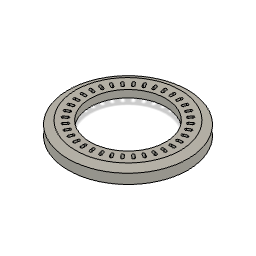
ROTORB (Autodesk Fusion 360 design; units mm, degrees)
Autodesk Fusion 360 part; units mm, degrees
sketch "Sketch1" plane through (0, 0, 0) normal (0, 1, 0) x (1, 0, 0)
  circle A0 centre (0, 0) radius 49.1
  dimension "d1" = 98.2
  constraint coincident A0.centre origin
  measures "d1" diameter of A0
ref_plane "WorkPlane1" through (0, 3, 0) normal (0, 1, 0) x (0, 0, 1)
sketch "Sketch2" plane through (0, 3, 0) normal (0, 1, 0) x (1, 0, 0)
  circle A0 centre (0, 0) radius 43
  dimension "d3" = 86
  constraint coincident A0.centre origin
  measures "d3" diameter of A0
loft "Loft1" add profiles "Sketch1", "Sketch2" section 1 section 2
sketch "Sketch3" plane through (0, 3, 0) normal (0, 1, 0) x (-1, 0, 0)
  circle A0 centre (0, 0) radius 43
  circle A1 centre (0, 0) radius 31
  dimension "d4" = 62
  constraint coincident A0.centre A1.centre
  measures "d4" diameter of A1
extrude "Extrude1" cut sketch "Sketch3" against normal blind 50 contours A1
sketch "Sketch4" plane through (0, 0, 0) normal (0, -1, 0) x (1, 0, 0)
  circle A0 centre (0, 0) radius 31
  circle A1 centre (0, 0) radius 49.1
  circle A2 centre (0, 0) radius 49.1
  constraint concentric A0 A2
extrude "Extrude2" add sketch "Sketch4" along normal blind 8
sketch "Sketch5" plane through (0, 3, 0) normal (0, 1, 0) x (-1, 0, 0)
  circle A0 centre (0, 0) radius 31
  circle A1 centre (0, 0) radius 43
  line L0 (-1, -35) -> (-1, -38)
  line L1 (1, -38) -> (1, -35)
  arc A2 (0, -39) -> (1, -38) centre (0, -38) ccw
  arc A3 (-1, -38) -> (0, -39) centre (0, -38) ccw
  arc A4 (0, -34) -> (-1, -35) centre (0, -35) ccw
  arc A5 (1, -35) -> (0, -34) centre (0, -35) ccw
  arc A6 (6.7723, -38.4075) -> (7.5834, -37.249) centre (6.5986, -37.4227) ccw
  arc A7 (7.0625, -34.2946) -> (5.904, -33.4835) centre (6.0777, -34.4683) ccw
  line L2 (7.5834, -37.249) -> (7.0625, -34.2946)
  arc A8 (5.904, -33.4835) -> (5.0929, -34.6419) centre (6.0777, -34.4683) ccw
  arc A9 (5.6138, -37.5963) -> (6.7723, -38.4075) centre (6.5986, -37.4227) ccw
  line L3 (5.0929, -34.6419) -> (5.6138, -37.5963)
  arc A10 (13.3388, -36.648) -> (13.9365, -35.3663) centre (12.9968, -35.7083) ccw
  arc A11 (12.9104, -32.5472) -> (11.6287, -31.9495) centre (11.9707, -32.8892) ccw
  line L4 (13.9365, -35.3663) -> (12.9104, -32.5472)
  arc A12 (11.6287, -31.9495) -> (11.031, -33.2313) centre (11.9707, -32.8892) ccw
  arc A13 (12.0571, -36.0503) -> (13.3388, -36.648) centre (12.9968, -35.7083) ccw
  line L5 (11.031, -33.2313) -> (12.0571, -36.0503)
  arc A14 (19.5, -33.775) -> (19.866, -32.409) centre (19, -32.909) ccw
  arc A15 (18.366, -29.8109) -> (17, -29.4449) centre (17.5, -30.3109) ccw
  line L6 (19.866, -32.409) -> (18.366, -29.8109)
  arc A16 (17, -29.4449) -> (16.634, -30.8109) centre (17.5, -30.3109) ccw
  arc A17 (18.134, -33.409) -> (19.5, -33.775) centre (19, -32.909) ccw
  line L7 (16.634, -30.8109) -> (18.134, -33.409)
  arc A18 (25.0687, -29.8757) -> (25.192, -28.4669) centre (24.4259, -29.1097) ccw
  arc A19 (23.2636, -26.1688) -> (21.8548, -26.0455) centre (22.4976, -26.8116) ccw
  line L8 (25.192, -28.4669) -> (23.2636, -26.1688)
  arc A20 (21.8548, -26.0455) -> (21.7315, -27.4543) centre (22.4976, -26.8116) ccw
  arc A21 (23.6599, -29.7525) -> (25.0687, -29.8757) centre (24.4259, -29.1097) ccw
  line L9 (21.7315, -27.4543) -> (23.6599, -29.7525)
  arc A22 (29.8757, -25.0687) -> (29.7525, -23.6599) centre (29.1097, -24.4259) ccw
  arc A23 (27.4543, -21.7315) -> (26.0455, -21.8548) centre (26.8116, -22.4976) ccw
  line L10 (29.7525, -23.6599) -> (27.4543, -21.7315)
  arc A24 (26.0455, -21.8548) -> (26.1688, -23.2636) centre (26.8116, -22.4976) ccw
  arc A25 (28.4669, -25.192) -> (29.8757, -25.0687) centre (29.1097, -24.4259) ccw
  line L11 (26.1688, -23.2636) -> (28.4669, -25.192)
  arc A26 (33.775, -19.5) -> (33.409, -18.134) centre (32.909, -19) ccw
  arc A27 (30.8109, -16.634) -> (29.4449, -17) centre (30.3109, -17.5) ccw
  line L12 (33.409, -18.134) -> (30.8109, -16.634)
  arc A28 (29.4449, -17) -> (29.8109, -18.366) centre (30.3109, -17.5) ccw
  arc A29 (32.409, -19.866) -> (33.775, -19.5) centre (32.909, -19) ccw
  line L13 (29.8109, -18.366) -> (32.409, -19.866)
  arc A30 (36.648, -13.3388) -> (36.0503, -12.0571) centre (35.7083, -12.9968) ccw
  arc A31 (33.2313, -11.031) -> (31.9495, -11.6287) centre (32.8892, -11.9707) ccw
  line L14 (36.0503, -12.0571) -> (33.2313, -11.031)
  arc A32 (31.9495, -11.6287) -> (32.5472, -12.9104) centre (32.8892, -11.9707) ccw
  arc A33 (35.3663, -13.9365) -> (36.648, -13.3388) centre (35.7083, -12.9968) ccw
  line L15 (32.5472, -12.9104) -> (35.3663, -13.9365)
  arc A34 (38.4075, -6.7723) -> (37.5963, -5.6138) centre (37.4227, -6.5986) ccw
  arc A35 (34.6419, -5.0929) -> (33.4835, -5.904) centre (34.4683, -6.0777) ccw
  line L16 (37.5963, -5.6138) -> (34.6419, -5.0929)
  arc A36 (33.4835, -5.904) -> (34.2946, -7.0625) centre (34.4683, -6.0777) ccw
  arc A37 (37.249, -7.5834) -> (38.4075, -6.7723) centre (37.4227, -6.5986) ccw
  line L17 (34.2946, -7.0625) -> (37.249, -7.5834)
  arc A38 (39, 0) -> (38, 1) centre (38, 0) ccw
  arc A39 (35, 1) -> (34, 0) centre (35, 0) ccw
  line L18 (38, 1) -> (35, 1)
  arc A40 (34, 0) -> (35, -1) centre (35, 0) ccw
  arc A41 (38, -1) -> (39, 0) centre (38, 0) ccw
  line L19 (35, -1) -> (38, -1)
  arc A42 (38.4075, 6.7723) -> (37.249, 7.5834) centre (37.4227, 6.5986) ccw
  arc A43 (34.2946, 7.0625) -> (33.4835, 5.904) centre (34.4683, 6.0777) ccw
  line L20 (37.249, 7.5834) -> (34.2946, 7.0625)
  arc A44 (33.4835, 5.904) -> (34.6419, 5.0929) centre (34.4683, 6.0777) ccw
  arc A45 (37.5963, 5.6138) -> (38.4075, 6.7723) centre (37.4227, 6.5986) ccw
  line L21 (34.6419, 5.0929) -> (37.5963, 5.6138)
  arc A46 (36.648, 13.3388) -> (35.3663, 13.9365) centre (35.7083, 12.9968) ccw
  arc A47 (32.5472, 12.9104) -> (31.9495, 11.6287) centre (32.8892, 11.9707) ccw
  line L22 (35.3663, 13.9365) -> (32.5472, 12.9104)
  arc A48 (31.9495, 11.6287) -> (33.2313, 11.031) centre (32.8892, 11.9707) ccw
  arc A49 (36.0503, 12.0571) -> (36.648, 13.3388) centre (35.7083, 12.9968) ccw
  line L23 (33.2313, 11.031) -> (36.0503, 12.0571)
  arc A50 (33.775, 19.5) -> (32.409, 19.866) centre (32.909, 19) ccw
  arc A51 (29.8109, 18.366) -> (29.4449, 17) centre (30.3109, 17.5) ccw
  line L24 (32.409, 19.866) -> (29.8109, 18.366)
  arc A52 (29.4449, 17) -> (30.8109, 16.634) centre (30.3109, 17.5) ccw
  arc A53 (33.409, 18.134) -> (33.775, 19.5) centre (32.909, 19) ccw
  line L25 (30.8109, 16.634) -> (33.409, 18.134)
  arc A54 (29.8757, 25.0687) -> (28.4669, 25.192) centre (29.1097, 24.4259) ccw
  arc A55 (26.1688, 23.2636) -> (26.0455, 21.8548) centre (26.8116, 22.4976) ccw
  line L26 (28.4669, 25.192) -> (26.1688, 23.2636)
  arc A56 (26.0455, 21.8548) -> (27.4543, 21.7315) centre (26.8116, 22.4976) ccw
  arc A57 (29.7525, 23.6599) -> (29.8757, 25.0687) centre (29.1097, 24.4259) ccw
  line L27 (27.4543, 21.7315) -> (29.7525, 23.6599)
  arc A58 (25.0687, 29.8757) -> (23.6599, 29.7525) centre (24.4259, 29.1097) ccw
  arc A59 (21.7315, 27.4543) -> (21.8548, 26.0455) centre (22.4976, 26.8116) ccw
  line L28 (23.6599, 29.7525) -> (21.7315, 27.4543)
  arc A60 (21.8548, 26.0455) -> (23.2636, 26.1688) centre (22.4976, 26.8116) ccw
  arc A61 (25.192, 28.4669) -> (25.0687, 29.8757) centre (24.4259, 29.1097) ccw
  line L29 (23.2636, 26.1688) -> (25.192, 28.4669)
  arc A62 (19.5, 33.775) -> (18.134, 33.409) centre (19, 32.909) ccw
  arc A63 (16.634, 30.8109) -> (17, 29.4449) centre (17.5, 30.3109) ccw
  line L30 (18.134, 33.409) -> (16.634, 30.8109)
  arc A64 (17, 29.4449) -> (18.366, 29.8109) centre (17.5, 30.3109) ccw
  arc A65 (19.866, 32.409) -> (19.5, 33.775) centre (19, 32.909) ccw
  line L31 (18.366, 29.8109) -> (19.866, 32.409)
  arc A66 (13.3388, 36.648) -> (12.0571, 36.0503) centre (12.9968, 35.7083) ccw
  arc A67 (11.031, 33.2313) -> (11.6287, 31.9495) centre (11.9707, 32.8892) ccw
  line L32 (12.0571, 36.0503) -> (11.031, 33.2313)
  arc A68 (11.6287, 31.9495) -> (12.9104, 32.5472) centre (11.9707, 32.8892) ccw
  arc A69 (13.9365, 35.3663) -> (13.3388, 36.648) centre (12.9968, 35.7083) ccw
  line L33 (12.9104, 32.5472) -> (13.9365, 35.3663)
  arc A70 (6.7723, 38.4075) -> (5.6138, 37.5963) centre (6.5986, 37.4227) ccw
  arc A71 (5.0929, 34.6419) -> (5.904, 33.4835) centre (6.0777, 34.4683) ccw
  line L34 (5.6138, 37.5963) -> (5.0929, 34.6419)
  arc A72 (5.904, 33.4835) -> (7.0625, 34.2946) centre (6.0777, 34.4683) ccw
  arc A73 (7.5834, 37.249) -> (6.7723, 38.4075) centre (6.5986, 37.4227) ccw
  line L35 (7.0625, 34.2946) -> (7.5834, 37.249)
  arc A74 (0, 39) -> (-1, 38) centre (0, 38) ccw
  arc A75 (-1, 35) -> (0, 34) centre (0, 35) ccw
  line L36 (-1, 38) -> (-1, 35)
  arc A76 (0, 34) -> (1, 35) centre (0, 35) ccw
  arc A77 (1, 38) -> (0, 39) centre (0, 38) ccw
  line L37 (1, 35) -> (1, 38)
  arc A78 (-6.7723, 38.4075) -> (-7.5834, 37.249) centre (-6.5986, 37.4227) ccw
  arc A79 (-7.0625, 34.2946) -> (-5.904, 33.4835) centre (-6.0777, 34.4683) ccw
  line L38 (-7.5834, 37.249) -> (-7.0625, 34.2946)
  arc A80 (-5.904, 33.4835) -> (-5.0929, 34.6419) centre (-6.0777, 34.4683) ccw
  arc A81 (-5.6138, 37.5963) -> (-6.7723, 38.4075) centre (-6.5986, 37.4227) ccw
  line L39 (-5.0929, 34.6419) -> (-5.6138, 37.5963)
  arc A82 (-13.3388, 36.648) -> (-13.9365, 35.3663) centre (-12.9968, 35.7083) ccw
  arc A83 (-12.9104, 32.5472) -> (-11.6287, 31.9495) centre (-11.9707, 32.8892) ccw
  line L40 (-13.9365, 35.3663) -> (-12.9104, 32.5472)
  arc A84 (-11.6287, 31.9495) -> (-11.031, 33.2313) centre (-11.9707, 32.8892) ccw
  arc A85 (-12.0571, 36.0503) -> (-13.3388, 36.648) centre (-12.9968, 35.7083) ccw
  line L41 (-11.031, 33.2313) -> (-12.0571, 36.0503)
  arc A86 (-19.5, 33.775) -> (-19.866, 32.409) centre (-19, 32.909) ccw
  arc A87 (-18.366, 29.8109) -> (-17, 29.4449) centre (-17.5, 30.3109) ccw
  line L42 (-19.866, 32.409) -> (-18.366, 29.8109)
  arc A88 (-17, 29.4449) -> (-16.634, 30.8109) centre (-17.5, 30.3109) ccw
  arc A89 (-18.134, 33.409) -> (-19.5, 33.775) centre (-19, 32.909) ccw
  line L43 (-16.634, 30.8109) -> (-18.134, 33.409)
  arc A90 (-25.0687, 29.8757) -> (-25.192, 28.4669) centre (-24.4259, 29.1097) ccw
  arc A91 (-23.2636, 26.1688) -> (-21.8548, 26.0455) centre (-22.4976, 26.8116) ccw
  line L44 (-25.192, 28.4669) -> (-23.2636, 26.1688)
  arc A92 (-21.8548, 26.0455) -> (-21.7315, 27.4543) centre (-22.4976, 26.8116) ccw
  arc A93 (-23.6599, 29.7525) -> (-25.0687, 29.8757) centre (-24.4259, 29.1097) ccw
  line L45 (-21.7315, 27.4543) -> (-23.6599, 29.7525)
  arc A94 (-29.8757, 25.0687) -> (-29.7525, 23.6599) centre (-29.1097, 24.4259) ccw
  arc A95 (-27.4543, 21.7315) -> (-26.0455, 21.8548) centre (-26.8116, 22.4976) ccw
  line L46 (-29.7525, 23.6599) -> (-27.4543, 21.7315)
  arc A96 (-26.0455, 21.8548) -> (-26.1688, 23.2636) centre (-26.8116, 22.4976) ccw
  arc A97 (-28.4669, 25.192) -> (-29.8757, 25.0687) centre (-29.1097, 24.4259) ccw
  line L47 (-26.1688, 23.2636) -> (-28.4669, 25.192)
  arc A98 (-33.775, 19.5) -> (-33.409, 18.134) centre (-32.909, 19) ccw
  arc A99 (-30.8109, 16.634) -> (-29.4449, 17) centre (-30.3109, 17.5) ccw
  line L48 (-33.409, 18.134) -> (-30.8109, 16.634)
  arc A100 (-29.4449, 17) -> (-29.8109, 18.366) centre (-30.3109, 17.5) ccw
  arc A101 (-32.409, 19.866) -> (-33.775, 19.5) centre (-32.909, 19) ccw
  line L49 (-29.8109, 18.366) -> (-32.409, 19.866)
  arc A102 (-36.648, 13.3388) -> (-36.0503, 12.0571) centre (-35.7083, 12.9968) ccw
  arc A103 (-33.2313, 11.031) -> (-31.9495, 11.6287) centre (-32.8892, 11.9707) ccw
  line L50 (-36.0503, 12.0571) -> (-33.2313, 11.031)
  arc A104 (-31.9495, 11.6287) -> (-32.5472, 12.9104) centre (-32.8892, 11.9707) ccw
  arc A105 (-35.3663, 13.9365) -> (-36.648, 13.3388) centre (-35.7083, 12.9968) ccw
  line L51 (-32.5472, 12.9104) -> (-35.3663, 13.9365)
  arc A106 (-38.4075, 6.7723) -> (-37.5963, 5.6138) centre (-37.4227, 6.5986) ccw
  arc A107 (-34.6419, 5.0929) -> (-33.4835, 5.904) centre (-34.4683, 6.0777) ccw
  line L52 (-37.5963, 5.6138) -> (-34.6419, 5.0929)
  arc A108 (-33.4835, 5.904) -> (-34.2946, 7.0625) centre (-34.4683, 6.0777) ccw
  arc A109 (-37.249, 7.5834) -> (-38.4075, 6.7723) centre (-37.4227, 6.5986) ccw
  line L53 (-34.2946, 7.0625) -> (-37.249, 7.5834)
  arc A110 (-39, 0) -> (-38, -1) centre (-38, 0) ccw
  arc A111 (-35, -1) -> (-34, 0) centre (-35, 0) ccw
  line L54 (-38, -1) -> (-35, -1)
  arc A112 (-34, 0) -> (-35, 1) centre (-35, 0) ccw
  arc A113 (-38, 1) -> (-39, 0) centre (-38, 0) ccw
  line L55 (-35, 1) -> (-38, 1)
  arc A114 (-38.4075, -6.7723) -> (-37.249, -7.5834) centre (-37.4227, -6.5986) ccw
  arc A115 (-34.2946, -7.0625) -> (-33.4835, -5.904) centre (-34.4683, -6.0777) ccw
  line L56 (-37.249, -7.5834) -> (-34.2946, -7.0625)
  arc A116 (-33.4835, -5.904) -> (-34.6419, -5.0929) centre (-34.4683, -6.0777) ccw
  arc A117 (-37.5963, -5.6138) -> (-38.4075, -6.7723) centre (-37.4227, -6.5986) ccw
  line L57 (-34.6419, -5.0929) -> (-37.5963, -5.6138)
  arc A118 (-36.648, -13.3388) -> (-35.3663, -13.9365) centre (-35.7083, -12.9968) ccw
  arc A119 (-32.5472, -12.9104) -> (-31.9495, -11.6287) centre (-32.8892, -11.9707) ccw
  line L58 (-35.3663, -13.9365) -> (-32.5472, -12.9104)
  arc A120 (-31.9495, -11.6287) -> (-33.2313, -11.031) centre (-32.8892, -11.9707) ccw
  arc A121 (-36.0503, -12.0571) -> (-36.648, -13.3388) centre (-35.7083, -12.9968) ccw
  line L59 (-33.2313, -11.031) -> (-36.0503, -12.0571)
  arc A122 (-33.775, -19.5) -> (-32.409, -19.866) centre (-32.909, -19) ccw
  arc A123 (-29.8109, -18.366) -> (-29.4449, -17) centre (-30.3109, -17.5) ccw
  line L60 (-32.409, -19.866) -> (-29.8109, -18.366)
  arc A124 (-29.4449, -17) -> (-30.8109, -16.634) centre (-30.3109, -17.5) ccw
  arc A125 (-33.409, -18.134) -> (-33.775, -19.5) centre (-32.909, -19) ccw
  line L61 (-30.8109, -16.634) -> (-33.409, -18.134)
  arc A126 (-29.8757, -25.0687) -> (-28.4669, -25.192) centre (-29.1097, -24.4259) ccw
  arc A127 (-26.1688, -23.2636) -> (-26.0455, -21.8548) centre (-26.8116, -22.4976) ccw
  line L62 (-28.4669, -25.192) -> (-26.1688, -23.2636)
  arc A128 (-26.0455, -21.8548) -> (-27.4543, -21.7315) centre (-26.8116, -22.4976) ccw
  arc A129 (-29.7525, -23.6599) -> (-29.8757, -25.0687) centre (-29.1097, -24.4259) ccw
  line L63 (-27.4543, -21.7315) -> (-29.7525, -23.6599)
  arc A130 (-25.0687, -29.8757) -> (-23.6599, -29.7525) centre (-24.4259, -29.1097) ccw
  arc A131 (-21.7315, -27.4543) -> (-21.8548, -26.0455) centre (-22.4976, -26.8116) ccw
  line L64 (-23.6599, -29.7525) -> (-21.7315, -27.4543)
  arc A132 (-21.8548, -26.0455) -> (-23.2636, -26.1688) centre (-22.4976, -26.8116) ccw
  arc A133 (-25.192, -28.4669) -> (-25.0687, -29.8757) centre (-24.4259, -29.1097) ccw
  line L65 (-23.2636, -26.1688) -> (-25.192, -28.4669)
  arc A134 (-19.5, -33.775) -> (-18.134, -33.409) centre (-19, -32.909) ccw
  arc A135 (-16.634, -30.8109) -> (-17, -29.4449) centre (-17.5, -30.3109) ccw
  line L66 (-18.134, -33.409) -> (-16.634, -30.8109)
  arc A136 (-17, -29.4449) -> (-18.366, -29.8109) centre (-17.5, -30.3109) ccw
  arc A137 (-19.866, -32.409) -> (-19.5, -33.775) centre (-19, -32.909) ccw
  line L67 (-18.366, -29.8109) -> (-19.866, -32.409)
  arc A138 (-13.3388, -36.648) -> (-12.0571, -36.0503) centre (-12.9968, -35.7083) ccw
  arc A139 (-11.031, -33.2313) -> (-11.6287, -31.9495) centre (-11.9707, -32.8892) ccw
  line L68 (-12.0571, -36.0503) -> (-11.031, -33.2313)
  arc A140 (-11.6287, -31.9495) -> (-12.9104, -32.5472) centre (-11.9707, -32.8892) ccw
  arc A141 (-13.9365, -35.3663) -> (-13.3388, -36.648) centre (-12.9968, -35.7083) ccw
  line L69 (-12.9104, -32.5472) -> (-13.9365, -35.3663)
  arc A142 (-6.7723, -38.4075) -> (-5.6138, -37.5963) centre (-6.5986, -37.4227) ccw
  arc A143 (-5.0929, -34.6419) -> (-5.904, -33.4835) centre (-6.0777, -34.4683) ccw
  line L70 (-5.6138, -37.5963) -> (-5.0929, -34.6419)
  arc A144 (-5.904, -33.4835) -> (-7.0625, -34.2946) centre (-6.0777, -34.4683) ccw
  arc A145 (-7.5834, -37.249) -> (-6.7723, -38.4075) centre (-6.5986, -37.4227) ccw
  line L71 (-7.0625, -34.2946) -> (-7.5834, -37.249)
  dimension "d9" = 1
  dimension "d11" = 360
  constraint tangent L1 A2
  constraint tangent L0 A3
  constraint equal A2 A3
  constraint coincident A2.start A3.end
  constraint tangent L0 A4
  constraint equal A2 A4
  constraint tangent L1 A5
  constraint equal A2 A5
  constraint coincident A4.start A5.end
  measures "d9" radius of A2
extrude "Extrude3" cut sketch "Sketch5" against normal blind 31 contours L0 L1 A2 A3 A4 A5 | A6 A7 L2 A8 A9 L3 | A10 A11 L4 A12 A13 L5 | A14 A15 L6 A16 A17 L7 | A18 A19 L8 A20 A21 L9 | A22 A23 L10 A24 A25 L11 | A26 A27 L12 A28 A29 L13 | A30 A31 L14 A32 A33 L15 | A34 A35 L16 A36 A37 L17 | A38 A39 L18 A40 A41 L19 | A42 A43 L20 A44 A45 L21 | A46 A47 L22 A48 A49 L23 | A50 A51 L24 A52 A53 L25 | A54 A55 L26 A56 A57 L27 | A58 A59 L28 A60 A61 L29 | A62 A63 L30 A64 A65 L31 | A66 A67 L32 A68 A69 L33 | A70 A71 L34 A72 A73 L35 | A74 A75 L36 A76 A77 L37 | A78 A79 L38 A80 A81 L39 | A82 A83 L40 A84 A85 L41 | A86 A87 L42 A88 A89 L43 | A90 A91 L44 A92 A93 L45 | A94 A95 L46 A96 A97 L47 | A98 A99 L48 A100 A101 L49 | A102 A103 L50 A104 A105 L51 | A106 A107 L52 A108 A109 L53 | A110 A111 L54 A112 A113 L55 | A114 A115 L56 A116 A117 L57 | A118 A119 L58 A120 A121 L59 | A122 A123 L60 A124 A125 L61 | A126 A127 L62 A128 A129 L63 | A130 A131 L64 A132 A133 L65 | A134 A135 L66 A136 A137 L67 | A138 A139 L68 A140 A141 L69 | A142 A143 L70 A144 A145 L71
sketch "Sketch6" plane through (0, -8, 0) normal (0, -1, 0) x (1, 0, 0)
  arc A0 (-13.9365, -35.3663) -> (-12.0571, -36.0503) centre (-12.9968, -35.7083) ccw
  line L0 (-13.9365, -35.3663) -> (-12.9104, -32.5472)
  arc A1 (-11.031, -33.2313) -> (-12.9104, -32.5472) centre (-11.9707, -32.8892) ccw
  line L1 (-11.031, -33.2313) -> (-12.0571, -36.0503)
  arc A2 (12.0571, -36.0503) -> (13.9365, -35.3663) centre (12.9968, -35.7083) ccw
  line L2 (12.0571, -36.0503) -> (11.031, -33.2313)
  arc A3 (12.9104, -32.5472) -> (11.031, -33.2313) centre (11.9707, -32.8892) ccw
  line L3 (12.9104, -32.5472) -> (13.9365, -35.3663)
  arc A4 (32.409, -19.866) -> (33.409, -18.134) centre (32.909, -19) ccw
  line L4 (32.409, -19.866) -> (29.8109, -18.366)
  arc A5 (30.8109, -16.634) -> (29.8109, -18.366) centre (30.3109, -17.5) ccw
  line L5 (30.8109, -16.634) -> (33.409, -18.134)
  arc A6 (37.5963, 5.6138) -> (37.249, 7.5834) centre (37.4227, 6.5986) ccw
  line L6 (37.5963, 5.6138) -> (34.6419, 5.0929)
  arc A7 (34.2946, 7.0625) -> (34.6419, 5.0929) centre (34.4683, 6.0777) ccw
  line L7 (34.2946, 7.0625) -> (37.249, 7.5834)
  arc A8 (25.192, 28.4669) -> (23.6599, 29.7525) centre (24.4259, 29.1097) ccw
  line L8 (25.192, 28.4669) -> (23.2636, 26.1688)
  arc A9 (21.7315, 27.4543) -> (23.2636, 26.1688) centre (22.4976, 26.8116) ccw
  line L9 (21.7315, 27.4543) -> (23.6599, 29.7525)
  arc A10 (1, 38) -> (-1, 38) centre (0, 38) ccw
  line L10 (1, 38) -> (1, 35)
  arc A11 (-1, 35) -> (1, 35) centre (0, 35) ccw
  line L11 (-1, 35) -> (-1, 38)
  arc A12 (-23.6599, 29.7525) -> (-25.192, 28.4669) centre (-24.4259, 29.1097) ccw
  line L12 (-23.6599, 29.7525) -> (-21.7315, 27.4543)
  arc A13 (-23.2636, 26.1688) -> (-21.7315, 27.4543) centre (-22.4976, 26.8116) ccw
  line L13 (-23.2636, 26.1688) -> (-25.192, 28.4669)
  arc A14 (-37.249, 7.5834) -> (-37.5963, 5.6138) centre (-37.4227, 6.5986) ccw
  line L14 (-37.249, 7.5834) -> (-34.2946, 7.0625)
  arc A15 (-34.6419, 5.0929) -> (-34.2946, 7.0625) centre (-34.4683, 6.0777) ccw
  line L15 (-34.6419, 5.0929) -> (-37.5963, 5.6138)
  arc A16 (-33.409, -18.134) -> (-32.409, -19.866) centre (-32.909, -19) ccw
  line L16 (-33.409, -18.134) -> (-30.8109, -16.634)
  arc A17 (-29.8109, -18.366) -> (-30.8109, -16.634) centre (-30.3109, -17.5) ccw
  line L17 (-29.8109, -18.366) -> (-32.409, -19.866)
  arc A18 (-36.0503, -12.0571) -> (-35.3663, -13.9365) centre (-35.7083, -12.9968) ccw
  line L18 (-36.0503, -12.0571) -> (-33.2313, -11.031)
  arc A19 (-32.5472, -12.9104) -> (-33.2313, -11.031) centre (-32.8892, -11.9707) ccw
  line L19 (-32.5472, -12.9104) -> (-35.3663, -13.9365)
  arc A20 (-35.3663, 13.9365) -> (-36.0503, 12.0571) centre (-35.7083, 12.9968) ccw
  line L20 (-35.3663, 13.9365) -> (-32.5472, 12.9104)
  arc A21 (-33.2313, 11.031) -> (-32.5472, 12.9104) centre (-32.8892, 11.9707) ccw
  line L21 (-33.2313, 11.031) -> (-36.0503, 12.0571)
  arc A22 (-18.134, 33.409) -> (-19.866, 32.409) centre (-19, 32.909) ccw
  line L22 (-18.134, 33.409) -> (-16.634, 30.8109)
  arc A23 (-18.366, 29.8109) -> (-16.634, 30.8109) centre (-17.5, 30.3109) ccw
  line L23 (-18.366, 29.8109) -> (-19.866, 32.409)
  arc A24 (7.5834, 37.249) -> (5.6138, 37.5963) centre (6.5986, 37.4227) ccw
  line L24 (7.5834, 37.249) -> (7.0625, 34.2946)
  arc A25 (5.0929, 34.6419) -> (7.0625, 34.2946) centre (6.0777, 34.4683) ccw
  line L25 (5.0929, 34.6419) -> (5.6138, 37.5963)
  arc A26 (29.7525, 23.6599) -> (28.4669, 25.192) centre (29.1097, 24.4259) ccw
  line L26 (29.7525, 23.6599) -> (27.4543, 21.7315)
  arc A27 (26.1688, 23.2636) -> (27.4543, 21.7315) centre (26.8116, 22.4976) ccw
  line L27 (26.1688, 23.2636) -> (28.4669, 25.192)
  arc A28 (38, -1) -> (38, 1) centre (38, 0) ccw
  line L28 (38, -1) -> (35, -1)
  arc A29 (35, 1) -> (35, -1) centre (35, 0) ccw
  line L29 (35, 1) -> (38, 1)
  arc A30 (28.4669, -25.192) -> (29.7525, -23.6599) centre (29.1097, -24.4259) ccw
  line L30 (28.4669, -25.192) -> (26.1688, -23.2636)
  arc A31 (27.4543, -21.7315) -> (26.1688, -23.2636) centre (26.8116, -22.4976) ccw
  line L31 (27.4543, -21.7315) -> (29.7525, -23.6599)
  arc A32 (5.6138, -37.5963) -> (7.5834, -37.249) centre (6.5986, -37.4227) ccw
  line L32 (5.6138, -37.5963) -> (5.0929, -34.6419)
  arc A33 (7.0625, -34.2946) -> (5.0929, -34.6419) centre (6.0777, -34.4683) ccw
  line L33 (7.0625, -34.2946) -> (7.5834, -37.249)
  arc A34 (-25.192, -28.4669) -> (-23.6599, -29.7525) centre (-24.4259, -29.1097) ccw
  line L34 (-25.192, -28.4669) -> (-23.2636, -26.1688)
  arc A35 (-21.7315, -27.4543) -> (-23.2636, -26.1688) centre (-22.4976, -26.8116) ccw
  line L35 (-21.7315, -27.4543) -> (-23.6599, -29.7525)
  arc A36 (-7.5834, -37.249) -> (-5.6138, -37.5963) centre (-6.5986, -37.4227) ccw
  line L36 (-7.5834, -37.249) -> (-7.0625, -34.2946)
  arc A37 (-5.0929, -34.6419) -> (-7.0625, -34.2946) centre (-6.0777, -34.4683) ccw
  line L37 (-5.0929, -34.6419) -> (-5.6138, -37.5963)
  arc A38 (18.134, -33.409) -> (19.866, -32.409) centre (19, -32.909) ccw
  line L38 (18.134, -33.409) -> (16.634, -30.8109)
  arc A39 (18.366, -29.8109) -> (16.634, -30.8109) centre (17.5, -30.3109) ccw
  line L39 (18.366, -29.8109) -> (19.866, -32.409)
  arc A40 (35.3663, -13.9365) -> (36.0503, -12.0571) centre (35.7083, -12.9968) ccw
  line L40 (35.3663, -13.9365) -> (32.5472, -12.9104)
  arc A41 (33.2313, -11.031) -> (32.5472, -12.9104) centre (32.8892, -11.9707) ccw
  line L41 (33.2313, -11.031) -> (36.0503, -12.0571)
  arc A42 (36.0503, 12.0571) -> (35.3663, 13.9365) centre (35.7083, 12.9968) ccw
  line L42 (36.0503, 12.0571) -> (33.2313, 11.031)
  arc A43 (32.5472, 12.9104) -> (33.2313, 11.031) centre (32.8892, 11.9707) ccw
  line L43 (32.5472, 12.9104) -> (35.3663, 13.9365)
  arc A44 (19.866, 32.409) -> (18.134, 33.409) centre (19, 32.909) ccw
  line L44 (19.866, 32.409) -> (18.366, 29.8109)
  arc A45 (16.634, 30.8109) -> (18.366, 29.8109) centre (17.5, 30.3109) ccw
  line L45 (16.634, 30.8109) -> (18.134, 33.409)
  arc A46 (-5.6138, 37.5963) -> (-7.5834, 37.249) centre (-6.5986, 37.4227) ccw
  line L46 (-5.6138, 37.5963) -> (-5.0929, 34.6419)
  arc A47 (-7.0625, 34.2946) -> (-5.0929, 34.6419) centre (-6.0777, 34.4683) ccw
  line L47 (-7.0625, 34.2946) -> (-7.5834, 37.249)
  arc A48 (-28.4669, 25.192) -> (-29.7525, 23.6599) centre (-29.1097, 24.4259) ccw
  line L48 (-28.4669, 25.192) -> (-26.1688, 23.2636)
  arc A49 (-27.4543, 21.7315) -> (-26.1688, 23.2636) centre (-26.8116, 22.4976) ccw
  line L49 (-27.4543, 21.7315) -> (-29.7525, 23.6599)
  arc A50 (-38, 1) -> (-38, -1) centre (-38, 0) ccw
  line L50 (-38, 1) -> (-35, 1)
  arc A51 (-35, -1) -> (-35, 1) centre (-35, 0) ccw
  line L51 (-35, -1) -> (-38, -1)
  arc A52 (-29.7525, -23.6599) -> (-28.4669, -25.192) centre (-29.1097, -24.4259) ccw
  line L52 (-29.7525, -23.6599) -> (-27.4543, -21.7315)
  arc A53 (-26.1688, -23.2636) -> (-27.4543, -21.7315) centre (-26.8116, -22.4976) ccw
  line L53 (-26.1688, -23.2636) -> (-28.4669, -25.192)
  arc A54 (-37.5963, -5.6138) -> (-37.249, -7.5834) centre (-37.4227, -6.5986) ccw
  line L54 (-37.5963, -5.6138) -> (-34.6419, -5.0929)
  arc A55 (-34.2946, -7.0625) -> (-34.6419, -5.0929) centre (-34.4683, -6.0777) ccw
  line L55 (-34.2946, -7.0625) -> (-37.249, -7.5834)
  arc A56 (-32.409, 19.866) -> (-33.409, 18.134) centre (-32.909, 19) ccw
  line L56 (-32.409, 19.866) -> (-29.8109, 18.366)
  arc A57 (-30.8109, 16.634) -> (-29.8109, 18.366) centre (-30.3109, 17.5) ccw
  line L57 (-30.8109, 16.634) -> (-33.409, 18.134)
  arc A58 (-12.0571, 36.0503) -> (-13.9365, 35.3663) centre (-12.9968, 35.7083) ccw
  line L58 (-12.0571, 36.0503) -> (-11.031, 33.2313)
  arc A59 (-12.9104, 32.5472) -> (-11.031, 33.2313) centre (-11.9707, 32.8892) ccw
  line L59 (-12.9104, 32.5472) -> (-13.9365, 35.3663)
  arc A60 (13.9365, 35.3663) -> (12.0571, 36.0503) centre (12.9968, 35.7083) ccw
  line L60 (13.9365, 35.3663) -> (12.9104, 32.5472)
  arc A61 (11.031, 33.2313) -> (12.9104, 32.5472) centre (11.9707, 32.8892) ccw
  line L61 (11.031, 33.2313) -> (12.0571, 36.0503)
  arc A62 (33.409, 18.134) -> (32.409, 19.866) centre (32.909, 19) ccw
  line L62 (33.409, 18.134) -> (30.8109, 16.634)
  arc A63 (29.8109, 18.366) -> (30.8109, 16.634) centre (30.3109, 17.5) ccw
  line L63 (29.8109, 18.366) -> (32.409, 19.866)
  arc A64 (37.249, -7.5834) -> (37.5963, -5.6138) centre (37.4227, -6.5986) ccw
  line L64 (37.249, -7.5834) -> (34.2946, -7.0625)
  arc A65 (34.6419, -5.0929) -> (34.2946, -7.0625) centre (34.4683, -6.0777) ccw
  line L65 (34.6419, -5.0929) -> (37.5963, -5.6138)
  arc A66 (23.6599, -29.7525) -> (25.192, -28.4669) centre (24.4259, -29.1097) ccw
  line L66 (23.6599, -29.7525) -> (21.7315, -27.4543)
  arc A67 (23.2636, -26.1688) -> (21.7315, -27.4543) centre (22.4976, -26.8116) ccw
  line L67 (23.2636, -26.1688) -> (25.192, -28.4669)
  line L68 (1, -35) -> (1, -38)
  arc A68 (-1, -38) -> (1, -38) centre (0, -38) ccw
  line L69 (-1, -38) -> (-1, -35)
  arc A69 (1, -35) -> (-1, -35) centre (0, -35) ccw
  arc A70 (-19.866, -32.409) -> (-18.134, -33.409) centre (-19, -32.909) ccw
  line L70 (-19.866, -32.409) -> (-18.366, -29.8109)
  arc A71 (-16.634, -30.8109) -> (-18.366, -29.8109) centre (-17.5, -30.3109) ccw
  line L71 (-16.634, -30.8109) -> (-18.134, -33.409)
  circle A72 centre (0, 0) radius 31
  circle A73 centre (0, 0) radius 49.1
  circle A74 centre (0, 0) radius 43.827
  circle A75 centre (0, 0) radius 41
  dimension "d14" = -5.273
  dimension "d15" = 82
  constraint coincident A72.centre A73.centre
  measures "d15" diameter of A75
extrude "Extrude4" cut sketch "Sketch6" against normal blind 5 contours A74
sketch "Sketch7" plane through (0, -8, 0) normal (0, -1, 0) x (1, 0, 0)
  circle A0 centre (0, 0) radius 41
  arc A1 (-13.9365, -35.3663) -> (-12.0571, -36.0503) centre (-12.9968, -35.7083) ccw
  line L0 (-13.9365, -35.3663) -> (-12.9104, -32.5472)
  arc A2 (-11.031, -33.2313) -> (-12.9104, -32.5472) centre (-11.9707, -32.8892) ccw
  line L1 (-11.031, -33.2313) -> (-12.0571, -36.0503)
  arc A3 (12.0571, -36.0503) -> (13.9365, -35.3663) centre (12.9968, -35.7083) ccw
  line L2 (12.0571, -36.0503) -> (11.031, -33.2313)
  arc A4 (12.9104, -32.5472) -> (11.031, -33.2313) centre (11.9707, -32.8892) ccw
  line L3 (12.9104, -32.5472) -> (13.9365, -35.3663)
  arc A5 (32.409, -19.866) -> (33.409, -18.134) centre (32.909, -19) ccw
  line L4 (32.409, -19.866) -> (29.8109, -18.366)
  arc A6 (30.8109, -16.634) -> (29.8109, -18.366) centre (30.3109, -17.5) ccw
  line L5 (30.8109, -16.634) -> (33.409, -18.134)
  arc A7 (37.5963, 5.6138) -> (37.249, 7.5834) centre (37.4227, 6.5986) ccw
  line L6 (37.5963, 5.6138) -> (34.6419, 5.0929)
  arc A8 (34.2946, 7.0625) -> (34.6419, 5.0929) centre (34.4683, 6.0777) ccw
  line L7 (34.2946, 7.0625) -> (37.249, 7.5834)
  arc A9 (25.192, 28.4669) -> (23.6599, 29.7525) centre (24.4259, 29.1097) ccw
  line L8 (25.192, 28.4669) -> (23.2636, 26.1688)
  arc A10 (21.7315, 27.4543) -> (23.2636, 26.1688) centre (22.4976, 26.8116) ccw
  line L9 (21.7315, 27.4543) -> (23.6599, 29.7525)
  arc A11 (1, 38) -> (-1, 38) centre (0, 38) ccw
  line L10 (1, 38) -> (1, 35)
  arc A12 (-1, 35) -> (1, 35) centre (0, 35) ccw
  line L11 (-1, 35) -> (-1, 38)
  arc A13 (-23.6599, 29.7525) -> (-25.192, 28.4669) centre (-24.4259, 29.1097) ccw
  line L12 (-23.6599, 29.7525) -> (-21.7315, 27.4543)
  arc A14 (-23.2636, 26.1688) -> (-21.7315, 27.4543) centre (-22.4976, 26.8116) ccw
  line L13 (-23.2636, 26.1688) -> (-25.192, 28.4669)
  arc A15 (-37.249, 7.5834) -> (-37.5963, 5.6138) centre (-37.4227, 6.5986) ccw
  line L14 (-37.249, 7.5834) -> (-34.2946, 7.0625)
  arc A16 (-34.6419, 5.0929) -> (-34.2946, 7.0625) centre (-34.4683, 6.0777) ccw
  line L15 (-34.6419, 5.0929) -> (-37.5963, 5.6138)
  arc A17 (-33.409, -18.134) -> (-32.409, -19.866) centre (-32.909, -19) ccw
  line L16 (-33.409, -18.134) -> (-30.8109, -16.634)
  arc A18 (-29.8109, -18.366) -> (-30.8109, -16.634) centre (-30.3109, -17.5) ccw
  line L17 (-29.8109, -18.366) -> (-32.409, -19.866)
  arc A19 (-36.0503, -12.0571) -> (-35.3663, -13.9365) centre (-35.7083, -12.9968) ccw
  line L18 (-36.0503, -12.0571) -> (-33.2313, -11.031)
  arc A20 (-32.5472, -12.9104) -> (-33.2313, -11.031) centre (-32.8892, -11.9707) ccw
  line L19 (-32.5472, -12.9104) -> (-35.3663, -13.9365)
  arc A21 (-35.3663, 13.9365) -> (-36.0503, 12.0571) centre (-35.7083, 12.9968) ccw
  line L20 (-35.3663, 13.9365) -> (-32.5472, 12.9104)
  arc A22 (-33.2313, 11.031) -> (-32.5472, 12.9104) centre (-32.8892, 11.9707) ccw
  line L21 (-33.2313, 11.031) -> (-36.0503, 12.0571)
  arc A23 (-18.134, 33.409) -> (-19.866, 32.409) centre (-19, 32.909) ccw
  line L22 (-18.134, 33.409) -> (-16.634, 30.8109)
  arc A24 (-18.366, 29.8109) -> (-16.634, 30.8109) centre (-17.5, 30.3109) ccw
  line L23 (-18.366, 29.8109) -> (-19.866, 32.409)
  arc A25 (7.5834, 37.249) -> (5.6138, 37.5963) centre (6.5986, 37.4227) ccw
  line L24 (7.5834, 37.249) -> (7.0625, 34.2946)
  arc A26 (5.0929, 34.6419) -> (7.0625, 34.2946) centre (6.0777, 34.4683) ccw
  line L25 (5.0929, 34.6419) -> (5.6138, 37.5963)
  arc A27 (29.7525, 23.6599) -> (28.4669, 25.192) centre (29.1097, 24.4259) ccw
  line L26 (29.7525, 23.6599) -> (27.4543, 21.7315)
  arc A28 (26.1688, 23.2636) -> (27.4543, 21.7315) centre (26.8116, 22.4976) ccw
  line L27 (26.1688, 23.2636) -> (28.4669, 25.192)
  arc A29 (38, -1) -> (38, 1) centre (38, 0) ccw
  line L28 (38, -1) -> (35, -1)
  arc A30 (35, 1) -> (35, -1) centre (35, 0) ccw
  line L29 (35, 1) -> (38, 1)
  arc A31 (28.4669, -25.192) -> (29.7525, -23.6599) centre (29.1097, -24.4259) ccw
  line L30 (28.4669, -25.192) -> (26.1688, -23.2636)
  arc A32 (27.4543, -21.7315) -> (26.1688, -23.2636) centre (26.8116, -22.4976) ccw
  line L31 (27.4543, -21.7315) -> (29.7525, -23.6599)
  arc A33 (5.6138, -37.5963) -> (7.5834, -37.249) centre (6.5986, -37.4227) ccw
  line L32 (5.6138, -37.5963) -> (5.0929, -34.6419)
  arc A34 (7.0625, -34.2946) -> (5.0929, -34.6419) centre (6.0777, -34.4683) ccw
  line L33 (7.0625, -34.2946) -> (7.5834, -37.249)
  arc A35 (-25.192, -28.4669) -> (-23.6599, -29.7525) centre (-24.4259, -29.1097) ccw
  line L34 (-25.192, -28.4669) -> (-23.2636, -26.1688)
  arc A36 (-21.7315, -27.4543) -> (-23.2636, -26.1688) centre (-22.4976, -26.8116) ccw
  line L35 (-21.7315, -27.4543) -> (-23.6599, -29.7525)
  arc A37 (-7.5834, -37.249) -> (-5.6138, -37.5963) centre (-6.5986, -37.4227) ccw
  line L36 (-7.5834, -37.249) -> (-7.0625, -34.2946)
  arc A38 (-5.0929, -34.6419) -> (-7.0625, -34.2946) centre (-6.0777, -34.4683) ccw
  line L37 (-5.0929, -34.6419) -> (-5.6138, -37.5963)
  arc A39 (18.134, -33.409) -> (19.866, -32.409) centre (19, -32.909) ccw
  line L38 (18.134, -33.409) -> (16.634, -30.8109)
  arc A40 (18.366, -29.8109) -> (16.634, -30.8109) centre (17.5, -30.3109) ccw
  line L39 (18.366, -29.8109) -> (19.866, -32.409)
  arc A41 (35.3663, -13.9365) -> (36.0503, -12.0571) centre (35.7083, -12.9968) ccw
  line L40 (35.3663, -13.9365) -> (32.5472, -12.9104)
  arc A42 (33.2313, -11.031) -> (32.5472, -12.9104) centre (32.8892, -11.9707) ccw
  line L41 (33.2313, -11.031) -> (36.0503, -12.0571)
  arc A43 (36.0503, 12.0571) -> (35.3663, 13.9365) centre (35.7083, 12.9968) ccw
  line L42 (36.0503, 12.0571) -> (33.2313, 11.031)
  arc A44 (32.5472, 12.9104) -> (33.2313, 11.031) centre (32.8892, 11.9707) ccw
  line L43 (32.5472, 12.9104) -> (35.3663, 13.9365)
  arc A45 (19.866, 32.409) -> (18.134, 33.409) centre (19, 32.909) ccw
  line L44 (19.866, 32.409) -> (18.366, 29.8109)
  arc A46 (16.634, 30.8109) -> (18.366, 29.8109) centre (17.5, 30.3109) ccw
  line L45 (16.634, 30.8109) -> (18.134, 33.409)
  arc A47 (-5.6138, 37.5963) -> (-7.5834, 37.249) centre (-6.5986, 37.4227) ccw
  line L46 (-5.6138, 37.5963) -> (-5.0929, 34.6419)
  arc A48 (-7.0625, 34.2946) -> (-5.0929, 34.6419) centre (-6.0777, 34.4683) ccw
  line L47 (-7.0625, 34.2946) -> (-7.5834, 37.249)
  arc A49 (-28.4669, 25.192) -> (-29.7525, 23.6599) centre (-29.1097, 24.4259) ccw
  line L48 (-28.4669, 25.192) -> (-26.1688, 23.2636)
  arc A50 (-27.4543, 21.7315) -> (-26.1688, 23.2636) centre (-26.8116, 22.4976) ccw
  line L49 (-27.4543, 21.7315) -> (-29.7525, 23.6599)
  arc A51 (-38, 1) -> (-38, -1) centre (-38, 0) ccw
  line L50 (-38, 1) -> (-35, 1)
  arc A52 (-35, -1) -> (-35, 1) centre (-35, 0) ccw
  line L51 (-35, -1) -> (-38, -1)
  arc A53 (-29.7525, -23.6599) -> (-28.4669, -25.192) centre (-29.1097, -24.4259) ccw
  line L52 (-29.7525, -23.6599) -> (-27.4543, -21.7315)
  arc A54 (-26.1688, -23.2636) -> (-27.4543, -21.7315) centre (-26.8116, -22.4976) ccw
  line L53 (-26.1688, -23.2636) -> (-28.4669, -25.192)
  arc A55 (-37.5963, -5.6138) -> (-37.249, -7.5834) centre (-37.4227, -6.5986) ccw
  line L54 (-37.5963, -5.6138) -> (-34.6419, -5.0929)
  arc A56 (-34.2946, -7.0625) -> (-34.6419, -5.0929) centre (-34.4683, -6.0777) ccw
  line L55 (-34.2946, -7.0625) -> (-37.249, -7.5834)
  arc A57 (-32.409, 19.866) -> (-33.409, 18.134) centre (-32.909, 19) ccw
  line L56 (-32.409, 19.866) -> (-29.8109, 18.366)
  arc A58 (-30.8109, 16.634) -> (-29.8109, 18.366) centre (-30.3109, 17.5) ccw
  line L57 (-30.8109, 16.634) -> (-33.409, 18.134)
  arc A59 (-12.0571, 36.0503) -> (-13.9365, 35.3663) centre (-12.9968, 35.7083) ccw
  line L58 (-12.0571, 36.0503) -> (-11.031, 33.2313)
  arc A60 (-12.9104, 32.5472) -> (-11.031, 33.2313) centre (-11.9707, 32.8892) ccw
  line L59 (-12.9104, 32.5472) -> (-13.9365, 35.3663)
  arc A61 (13.9365, 35.3663) -> (12.0571, 36.0503) centre (12.9968, 35.7083) ccw
  line L60 (13.9365, 35.3663) -> (12.9104, 32.5472)
  arc A62 (11.031, 33.2313) -> (12.9104, 32.5472) centre (11.9707, 32.8892) ccw
  line L61 (11.031, 33.2313) -> (12.0571, 36.0503)
  arc A63 (33.409, 18.134) -> (32.409, 19.866) centre (32.909, 19) ccw
  line L62 (33.409, 18.134) -> (30.8109, 16.634)
  arc A64 (29.8109, 18.366) -> (30.8109, 16.634) centre (30.3109, 17.5) ccw
  line L63 (29.8109, 18.366) -> (32.409, 19.866)
  arc A65 (37.249, -7.5834) -> (37.5963, -5.6138) centre (37.4227, -6.5986) ccw
  line L64 (37.249, -7.5834) -> (34.2946, -7.0625)
  arc A66 (34.6419, -5.0929) -> (34.2946, -7.0625) centre (34.4683, -6.0777) ccw
  line L65 (34.6419, -5.0929) -> (37.5963, -5.6138)
  arc A67 (23.6599, -29.7525) -> (25.192, -28.4669) centre (24.4259, -29.1097) ccw
  line L66 (23.6599, -29.7525) -> (21.7315, -27.4543)
  arc A68 (23.2636, -26.1688) -> (21.7315, -27.4543) centre (22.4976, -26.8116) ccw
  line L67 (23.2636, -26.1688) -> (25.192, -28.4669)
  line L68 (1, -35) -> (1, -38)
  arc A69 (-1, -38) -> (1, -38) centre (0, -38) ccw
  line L69 (-1, -38) -> (-1, -35)
  arc A70 (1, -35) -> (-1, -35) centre (0, -35) ccw
  arc A71 (-19.866, -32.409) -> (-18.134, -33.409) centre (-19, -32.909) ccw
  line L70 (-19.866, -32.409) -> (-18.366, -29.8109)
  arc A72 (-16.634, -30.8109) -> (-18.366, -29.8109) centre (-17.5, -30.3109) ccw
  line L71 (-16.634, -30.8109) -> (-18.134, -33.409)
  circle A73 centre (0, 0) radius 31
  circle A74 centre (0, 0) radius 41
  constraint coincident A0.centre A73.centre
extrude "Extrude5" cut sketch "Sketch7" against normal blind 5 contours A0 A74 | A1 L0 A2 L1 | A3 L2 A4 L3 | A5 L4 A6 L5 | A7 L6 A8 L7 | A9 L8 A10 L9 | A11 L10 A12 L11 | A13 L12 A14 L13 | A15 L14 A16 L15 | A17 L16 A18 L17 | A19 L18 A20 L19 | A21 L20 A22 L21 | A23 L22 A24 L23 | A25 L24 A26 L25 | A27 L26 A28 L27 | A29 L28 A30 L29 | A31 L30 A32 L31 | A33 L32 A34 L33 | A35 L34 A36 L35 | A37 L36 A38 L37 | A39 L38 A40 L39 | A41 L40 A42 L41 | A43 L42 A44 L43 | A45 L44 A46 L45 | A47 L46 A48 L47 | A49 L48 A50 L49 | A51 L50 A52 L51 | A53 L52 A54 L53 | A55 L54 A56 L55 | A57 L56 A58 L57 | A59 L58 A60 L59 | A61 L60 A62 L61 | A63 L62 A64 L63 | A65 L64 A66 L65 | A67 L66 A68 L67 | L68 A69 L69 A70 | A71 L70 A72 L71 | A73
thread "Thread1" "ISO Metric profile 95.0 M95x2 6H" major diameter 95.2695 minor diameter 93.0225 pitch 2 angle 60 resizes the face on face at (43.7725, -4.6667, -2.1846)
